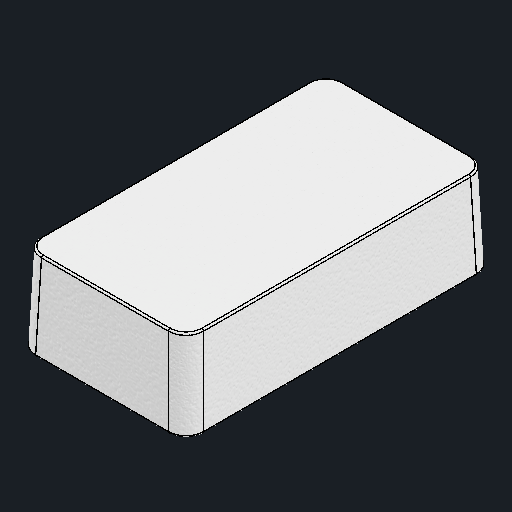
# Autodesk Inventor part: Compressor
Saved by Autodesk Inventor 2026.2 (Build 302298000, 298)
## iProperties
Created: 2026-05-18
Part Number: Compressor
Material: Aluminum 6061
Document SubType Name: Modeling
Designer: JoshuaEah
Density: 2.7 g/cm^3
Appearance: Coarse Textured - White
Author: JoshuaEah
Autodesk Inventor part; units mm, degrees
ref_plane "YZ Plane" through (0, 0, 0) normal (1, 0, 0) x (0, 1, 0)
ref_plane "XZ Plane" through (0, 0, 0) normal (0, 1, 0) x (-1, 0, 0)
ref_plane "XY Plane" through (0, 0, 0) normal (0, 0, 1) x (1, 0, 0)
sketch "Sketch1" plane through (0, 0, 0) normal (0, 1, 0) x (-1, 0, 0)
  line L0 (0, 0) -> (-60.96, 0)
  line L1 (-60.96, 0) -> (-60.96, -111.76)
  line L2 (-60.96, -111.76) -> (0, -111.76)
  line L3 (0, -111.76) -> (0, 0)
  dimension "d0" = 60.96
  dimension "d1" = 111.76
  constraints: 8 end point, 2 parallel, 1 coincident, 1 horizontal, 1 perpendicular
  measures "d0" distance of L2.end L1.end
  measures "d1" distance of L1.end L0.end
extrude "Extrusion1" add sketch "Sketch1" along normal blind 31.75 draft -2
fillet "Fillet1" radius 6.35 4 edges at (60.4056, 15.875, -0.5544) (60.4056, 15.875, -111.2056) (0.5544, 15.875, -111.2056) (0.5544, 15.875, -0.5544)
fillet "Fillet2" radius 0.635 16 edges at (57.993, 31.75, -2.967) (30.48, 31.75, -1.1087) (2.967, 31.75, -2.967) (1.1087, 31.75, -55.88) (2.967, 31.75, -108.793) (30.48, 31.75, -110.6513) (57.993, 31.75, -108.793) (59.8513, 31.75, -55.88) (59.1017, 0, -109.9017) (30.48, 0, -111.76) (1.8583, 0, -109.9017) (0, 0, -55.88) (1.8583, 0, -1.8583) (30.48, 0, 0) (59.1017, 0, -1.8583) (60.96, 0, -55.88)
body "Solid1"
